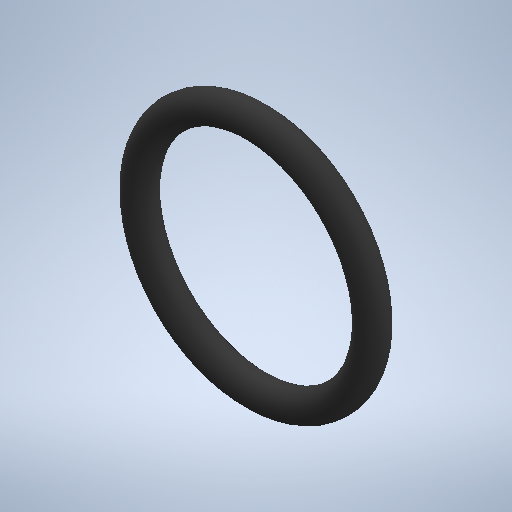
# Autodesk Inventor part: O-ring_D63
Saved by Autodesk Inventor 2025.3 (Build 293356030, 356C)
## iProperties
Created: 2025-09-06
Part Number: O-ring_D63
Material: 一般
Document SubType Name: Modeling
Designer: daisuke
Density: 1 g/cm^3
Appearance: ゴム - 黒
Author: daisuke
Autodesk Inventor part; units mm, degrees
ref_plane "YZ Plane" through (0, 0, 0) normal (1, 0, 0) x (0, 1, 0)
ref_plane "XZ Plane" through (0, 0, 0) normal (0, 1, 0) x (-1, 0, 0)
ref_plane "XY Plane" through (0, 0, 0) normal (0, 0, 1) x (1, 0, 0)
sketch "スケッチ1" plane through (0, 0, 0) normal (0, 1, 0) x (-1, 0, 0)
  line L0 (0, 0) -> (-88.8094, 0) construction
  circle A0 centre (0, 0) radius 12.35 construction
  circle A1 centre (0, 0) radius 15.85 construction
  line L1 (-15.85, -14.3346) -> (-15.85, 14.3346) construction
  line L2 (-14.1, 17.2911) -> (-14.1, -17.2911) construction
  line L3 (-12.35, -14.4815) -> (-12.35, 14.4815) construction
  circle A2 centre (-14.1, 0) radius 1.75
  line L4 (0, -24.2075) -> (0, 24.2075) projected
  point P0 (-15.85, 0)
  point P1 (-12.35, 0)
  dimension "IN_D" = 24.7
  dimension "W_D" = 3.5
  constraints: 8 end point, 3 centre point, 3 coincident, 3 midpoint, 3 point on line, 3 tangent, 2 vertical, 1 horizontal, 1 other
  measures "IN_D" diameter of A0
  measures "W_D" diameter of A2
revolve "回転1" add sketch "スケッチ1" angle 360 about axis through (0, 0, -10) along (0, 0, 1)
